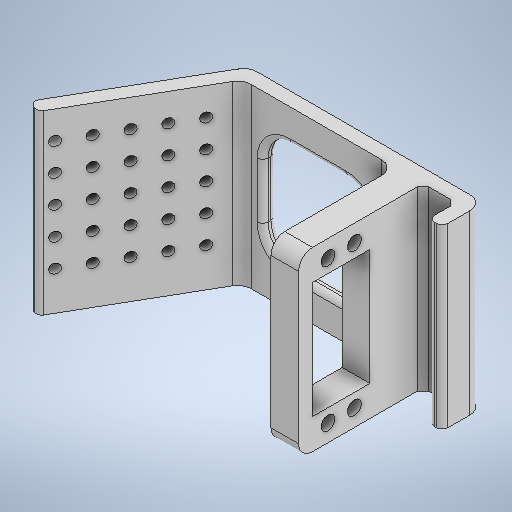
# Autodesk Inventor part: Support2
Saved by Autodesk Inventor 2025 (Build 290162000, 162)
## iProperties
Created: 2024-04-07
Part Number: Support2
Material: Générique
Document SubType Name: Modeling
Designer: chass
Density: 1 g/cm^3
Appearance: Par défaut
Author: chass
## iProperties of the stored document Support2_Impression 3D.ipt
Created: 2024-04-07
Part Number: Support2_Impression 3D
Material: Générique
Document SubType Name: Modeling
Designer: chass
Density: 1 g/cm^3
Appearance: Par défaut
Author: chass
Autodesk Inventor part; units mm, degrees
ref_plane "YZ Plane" through (0, 0, 0) normal (1, 0, 0) x (0, 1, 0)
ref_plane "XZ Plane" through (0, 0, 0) normal (0, 1, 0) x (-1, 0, 0)
ref_plane "XY Plane" through (0, 0, 0) normal (0, 0, 1) x (1, 0, 0)
sketch "Esquisse1" plane through (0, 0, 0) normal (1, 0, 0) x (0, 1, 0)
  line L0 (32, 15.4) -> (-32, 15.4)
  line L1 (-32, 15.4) -> (-32, -34.6)
  line L2 (-32, -34.6) -> (32, -34.6)
  line L3 (32, -34.6) -> (32, 15.4)
  line L4 (21, 10.4) -> (-21, 10.4)
  line L5 (-21, 10.4) -> (-21, -10.4)
  line L6 (-21, -10.4) -> (21, -10.4)
  line L7 (21, -10.4) -> (21, 10.4)
  line L8 (21, 10.4) -> (-21, -10.4)
  line L9 (-21, 10.4) -> (21, -10.4)
  circle A0 centre (25.791, 4.75) radius 2.5
  circle A1 centre (25.791, -4.75) radius 2.5
  line L10 (0, 10.4) -> (0, -10.4)
  circle A2 centre (-25.791, 4.75) radius 2.5
  circle A3 centre (-25.791, -4.75) radius 2.5
  point P0 (0, 0)
  point P1 (0, 0)
  point P2 (0, 0)
  point P3 (0, 0)
  point P4 (0, 0)
  dimension "d0" = 50
  dimension "d1" = 64
  dimension "d2" = 42
  dimension "d3" = 20.8
  dimension "d4" = 5
  dimension "d5" = 4.791
  dimension "d69" = 5
  constraints: 22 end point, 4 centre point, 4 midpoint, 4 parallel, 3 coincident, 2 horizontal, 2 perpendicular, 2 symmetric about line, 2 other
  measures "d0" distance of L2.end L0.start
  measures "d1" distance of L0.start L0.end
  measures "d2" distance of L5.end L6.end
  measures "d3" distance of L6.end L4.start
  measures "d4" diameter of A0
  measures "d5" distance from line of L7 A0.centre
  measures "d69" distance between parallel lines of L0 L4
extrude "Extrusion1" add sketch "Esquisse1" along normal blind 10
sketch "Esquisse2" plane through (10, 0, 0) normal (1, 0, 0) x (0, 0, -1)
  line L0 (-10.4, -21) -> (-10.4, 21) projected
  line L1 (-15.4, -32) -> (6.7, -32)
  line L2 (0, -32) -> (0, 32)
  line L3 (15.4, -32) -> (-34.6, -32)
  line L4 (34.6, -32) -> (34.6, 32) projected
  line L5 (34.6, 32) -> (29.6, 32)
  line L6 (29.6, 32) -> (29.6, -32)
  line L7 (29.6, -32) -> (34.6, -32)
  line L8 (34.6, -32) -> (34.6, 32)
  point P0 (0, 0)
  dimension "d66" = 5
  constraints: 14 end point, 2 horizontal, 2 parallel, 2 symmetric about line, 1 perpendicular, 1 point on line, 1 vertical, 1 other
  measures "d66" distance of L7.end L6.end
extrude "Extrusion2" add sketch "Esquisse2" along normal blind 17
sketch "Esquisse4" plane through (0, 0, 0) normal (-1, 0, 0) x (0, 0, 1)
  line L0 (-34.6, -32) -> (-34.6, 32) projected
  line L1 (15.4, -32) -> (-34.6, -32) projected
  line L2 (-34.6, 32) -> (-29.6, 32)
  line L3 (-29.6, 32) -> (-29.6, -32)
  line L4 (-29.6, -32) -> (-34.6, -32)
  line L5 (-34.6, -32) -> (-34.6, 32)
  point P0 (0, 0)
  dimension "d14" = 5
  constraints: 8 end point, 2 parallel, 1 horizontal, 1 perpendicular, 1 point on line
  measures "d14" distance of L3.end L4.end
extrude "Extrusion4" add sketch "Esquisse4" along normal blind 55
sketch "Esquisse5" plane through (0, 32, 15.4) normal (0, 1, 0) x (1, 0, 0)
  line L0 (0, 45) -> (-55, 45) projected
  line L1 (-55, 45) -> (-82.4241, -2.5)
  line L2 (-55, 45) -> (-0.1517, 45) construction
  line L3 (-82.4241, -2.5) -> (-86.7543, 0)
  line L4 (-86.7543, 0) -> (-57.8868, 50)
  line L5 (-55, 50) -> (27, 50) projected
  line L6 (-57.8868, 50) -> (-55, 50)
  line L7 (-55, 45) -> (-55, 50)
  point P0 (0, 15.4)
  point P1 (25, 65)
  point P2 (10, 65)
  point P3 (23, 50)
  dimension "d17" = 120
  dimension "d18" = 5
  dimension "d19" = 90
  dimension "d53" = 50
  constraints: 12 end point, 2 horizontal, 1 equal length, 1 perpendicular, 1 vertical, 1 other
  measures "d17" angle of L1 L2
  measures "d18" distance of L1.end L3.end
  measures "d19" angle of L3 L4
  measures "d53" vertical distance of L3.end L4.end
extrude "Extrusion5" add sketch "Esquisse5" against normal blind 64
sketch "Esquisse6" plane through (-57.8868, -32, -34.6) normal (-0.8660254, 0, -0.5) x (-0.5, 0, 0.8660254)
  circle A0 centre (12.735, 54) radius 1.75
  line L0 (12.735, 54) -> (22.735, 54)
  circle A1 centre (22.735, 54) radius 1.75
  line L1 (22.735, 54) -> (32.735, 54)
  circle A2 centre (32.735, 54) radius 1.75
  line L2 (0, 64) -> (0, 0) projected
  line L3 (56, 0) -> (0, 0)
  circle A3 centre (52.735, 54) radius 1.75
  circle A4 centre (42.735, 54) radius 1.75
  line L4 (10.985, 49) -> (54.485, 49)
  line L5 (10.985, 49) -> (54.485, 49) construction
  circle A5 centre (12.735, 44) radius 1.75
  circle A6 centre (22.735, 44) radius 1.75
  circle A7 centre (32.735, 44) radius 1.75
  circle A8 centre (52.735, 44) radius 1.75
  circle A9 centre (42.735, 44) radius 1.75
  line L6 (10.985, 39) -> (54.485, 39)
  circle A10 centre (12.735, 24) radius 1.75
  line L7 (12.735, 24) -> (22.735, 24)
  circle A11 centre (22.735, 24) radius 1.75
  line L8 (22.735, 24) -> (32.735, 24)
  circle A12 centre (32.735, 24) radius 1.75
  circle A13 centre (52.735, 24) radius 1.75
  circle A14 centre (42.735, 24) radius 1.75
  line L9 (10.985, 29) -> (54.485, 29)
  line L10 (10.985, 29) -> (54.485, 29) construction
  circle A15 centre (12.735, 34) radius 1.75
  circle A16 centre (22.735, 34) radius 1.75
  circle A17 centre (32.735, 34) radius 1.75
  circle A18 centre (42.735, 34) radius 1.75
  circle A19 centre (52.735, 34) radius 1.75
  line L11 (10.985, 19) -> (54.485, 19)
  circle A20 centre (32.735, 14) radius 1.75
  line L12 (22.735, 14) -> (32.735, 14)
  line L13 (12.735, 14) -> (22.735, 14)
  circle A21 centre (12.735, 14) radius 1.75
  circle A22 centre (22.735, 14) radius 1.75
  circle A23 centre (42.735, 14) radius 1.75
  circle A24 centre (52.735, 14) radius 1.75
  line L14 (0, 64) -> (57.735, 64) projected
  line L15 (57.735, 64) -> (57.735, 0) projected
  dimension "d41" = 3.5
  dimension "d42" = 3.5
  dimension "d43" = 10
  dimension "d44" = 10
  dimension "d45" = 3.5
  dimension "d47" = 5
  dimension "d48" = 5
  dimension "d49" = 5
  dimension "d71" = 5
  dimension "d72" = 10
  dimension "d73" = 10
  constraints: 27 symmetric about line, 26 end point, 25 centre point, 6 coincident, 5 horizontal, 1 collinear, 1 perpendicular, 20 other
  measures "d41" diameter of A0
  measures "d42" diameter of A1
  measures "d43" distance of L0.start L0.end
  measures "d44" distance of L1.start L1.end
  measures "d45" diameter of A2
  measures "d47" distance from line of L4 L1.end
  measures "d48" distance from line of L6 A7.centre
  measures "d49" distance from line of L11 A12.centre
  measures "d71" distance from line of L15 A3.centre
  measures "d72" distance of A3.centre A4.centre
  measures "d73" distance of A4.centre L1.end
extrude "Extrusion6" cut sketch "Esquisse6" against normal blind 10
fillet "Congé de faces1" radius 5 1 edges at (-55, 0, -29.6)
fillet "Congé de faces2" radius 5 1 edges at (0, 0, -29.6)
fillet "Congé de faces3" radius 5 1 edges at (-57.8868, 0, -34.6)
sketch "Esquisse8" plane through (10, -32, -29.6) normal (0, 0, 1) x (1, 0, 0)
  line L0 (17, 64) -> (17, 0) projected
  line L1 (0, 0) -> (17, 0) projected
  line L2 (17, 64) -> (12, 64)
  line L3 (12, 64) -> (12, 0)
  line L4 (12, 0) -> (17, 0)
  line L5 (17, 0) -> (17, 64)
  point P0 (-10, 32)
  dimension "d76" = 5
  constraints: 8 end point, 2 parallel, 1 horizontal, 1 perpendicular, 1 point on line
  measures "d76" distance of L0.start L2.end
extrude "Extrusion8" add sketch "Esquisse8" along normal blind 10
fillet "Congé4" radius 5 1 edges at (27, 0, -34.6)
fillet "Congé5" radius 5 2 edges at (5, -32, 15.4) (5, 32, 15.4)
fillet "Congé6" radius 2 2 edges at (22, 0, -19.6) (27, 0, -19.6)
chamfer "Chanfrein1" distance 2 angle 45 2 edges at (10, 0, -29.6) (22, 0, -29.6)
fillet "Congé7" radius 2 2 edges at (-86.7543, 0, 15.4) (-82.4241, 0, 17.9)
sketch "Esquisse9" plane through (-55, -32, -34.6) normal (0, 0, -1) x (-1, 0, 0)
  line L0 (-47, 52) -> (-7, 52)
  line L1 (-7, 52) -> (-7, 12)
  line L2 (-7, 12) -> (-47, 12)
  line L3 (-47, 12) -> (-47, 52)
  line L4 (0, 0) -> (-77, 0) projected
  line L5 (-82, 64) -> (-82, 0) projected
  point P0 (-55, 32)
  dimension "d84" = 40
  dimension "d85" = 40
  dimension "d86" = 12
  dimension "d88" = 35
  constraints: 8 end point, 2 parallel, 1 horizontal, 1 perpendicular
  measures "d84" distance of L2.end L0.start
  measures "d85" distance of L0.start L0.end
  measures "d86" distance between parallel lines of L4 L2
  measures "d88" distance between parallel lines of L5 L3
extrude "Extrusion9" cut sketch "Esquisse9" against normal blind 17
fillet "Congé9" radius 10 4 edges at (-48, 20, -32.1) (-8, 20, -32.1) (-8, -20, -32.1) (-48, -20, -32.1)
fillet "Congé10" radius 2 16 edges at (-10.9289, -17.0711, -34.6) (-8, 0, -34.6) (-10.9289, 17.0711, -34.6) (-28, 20, -34.6) (-45.0711, 17.0711, -34.6) (-48, 0, -34.6) (-45.0711, -17.0711, -34.6) (-28, -20, -34.6) (-45.0711, -17.0711, -29.6) (-48, 0, -29.6) (-45.0711, 17.0711, -29.6) (-28, 20, -29.6) (-10.9289, 17.0711, -29.6) (-8, 0, -29.6) (-10.9289, -17.0711, -29.6) (-28, -20, -29.6)
